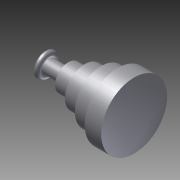
# Autodesk Inventor part: lesson4
Saved by Autodesk Inventor 2012 (Build 160160000, 160)
## iProperties
Created: 2011-10-08
Part Number: lesson4
Document SubType Name: Modeling
Designer: Kevin
Density: 1 g/cm^3
Material: Default
Author: Kevin
Autodesk Inventor part; units mm, degrees
ref_plane "YZ Plane" through (0, 0, 0) normal (1, 0, 0) x (0, 1, 0)
ref_plane "XZ Plane" through (0, 0, 0) normal (0, 1, 0) x (-1, 0, 0)
ref_plane "XY Plane" through (0, 0, 0) normal (0, 0, 1) x (1, 0, 0)
sketch "Sketch1" plane through (0, 0, 0) normal (0, 0, 1) x (1, 0, 0)
  line L0 (-42.6611, 7.6335) -> (42.1293, 7.6335) construction
  line L1 (25.6024, 7.6335) -> (25.6024, 17.6335)
  line L2 (25.6024, 17.6335) -> (20.6024, 17.6335)
  line L3 (20.6024, 17.6335) -> (20.6024, 15.6335)
  line L4 (20.6024, 15.6335) -> (15.6024, 15.6335)
  line L5 (15.6024, 15.6335) -> (15.6024, 13.6335)
  line L6 (15.6024, 13.6335) -> (10.6024, 13.6335)
  line L7 (10.6024, 13.6335) -> (10.6024, 11.6335)
  line L8 (10.6024, 11.6335) -> (5.6024, 11.6335)
  line L9 (5.6024, 11.6335) -> (5.6024, 9.6335)
  line L10 (5.6024, 9.6335) -> (-0.3976, 9.6335)
  arc A0 (-0.3976, 9.6335) -> (-1.1976, 11.2335) centre (-1.1976, 10.2335) ccw
  line L11 (-1.1976, 10.2335) -> (-1.1976, 7.6335)
  line L12 (-1.1976, 10.2335) -> (-1.1976, 11.2335)
  line L13 (-1.1976, 7.6335) -> (25.6024, 7.6335)
  point P0 (0, 0)
  dimension "d2" = 5
  dimension "d3" = 5
  dimension "d4" = 5
  dimension "d5" = 5
  dimension "d7" = 2
  dimension "d8" = 2
  dimension "d9" = 2
  dimension "d10" = 2
  dimension "d11" = 2
  dimension "d12" = 2
  constraints: 28 end point, 7 parallel, 4 perpendicular, 2 point on circle, 2 point on line, 1 centre point, 1 collinear, 1 horizontal
  measures "d2" distance of L1.end L2.end
  measures "d3" distance of L3.end L4.end
  measures "d4" distance of L5.end L6.end
  measures "d5" distance of L7.end L8.end
  measures "d7" distance between parallel lines of L0 L10
  measures "d8" distance of L8.end L9.end
  measures "d9" distance of L6.end L7.end
  measures "d10" distance of L4.end L5.end
  measures "d11" distance of L2.end L3.end
  measures "d12" diameter of A0
revolve "Revolution1" add sketch "Sketch1" angle 360 about axis through (-42.6611, 7.6335, 0) along (1, 0, 0)
body "Solid1"
